Autodesk Inventor part; units mm, degrees
(part 4 of 4)
  line L290 (119.5666, 122.9451) -> (119.5666, 123.8935)
  line L291 (119.5666, 123.8935) -> (127.8065, 123.8935)
  line L292 (127.8065, 123.8935) -> (127.8065, 125.5163)
  line L293 (127.8065, 125.5163) -> (128.7402, 125.5163)
  line L294 (128.7402, 126.4722) -> (119.5962, 129.5548)
  line L295 (119.5962, 129.5548) -> (119.5962, 131.0516)
  line L296 (119.5962, 131.0516) -> (128.7402, 134.1342)
  line L297 (128.7402, 134.1342) -> (128.7402, 132.8523)
  line L298 (128.7402, 132.8523) -> (126.1837, 132.0224)
  line L299 (126.1837, 132.0224) -> (126.1837, 128.5322)
  line L300 (126.1837, 128.5322) -> (128.7402, 127.7023)
  line L301 (128.7402, 127.7023) -> (128.7402, 126.4722)
  line L302 (125.1463, 131.6889) -> (120.8411, 130.2736)
  line L303 (120.8411, 130.2736) -> (125.1463, 128.8657)
  line L304 (125.1463, 128.8657) -> (125.1463, 131.6889)
  spline S260 degree 2 poles (128.9032, 141.4776) (128.9032, 140.4846) (128.4883, 139.0916) (128.1919, 138.4765) knots 0 0 0 1 2 2 2
  line L305 (128.1919, 138.4765) -> (126.6654, 138.4765)
  line L306 (126.6654, 138.4765) -> (126.6654, 138.5654)
  spline S261 degree 2 poles (126.6654, 138.5654) (127.2286, 139.1657) (127.851, 140.6847) (127.851, 141.3887) knots 0 0 0 1 2 2 2
  spline S262 degree 2 poles (127.851, 141.3887) (127.851, 142.3964) (127.0137, 143.4264) (126.3245, 143.4264) knots 0 0 0 1 2 2 2
  spline S263 degree 2 poles (126.3245, 143.4264) (125.7762, 143.4264) (125.0945, 142.8855) (124.924, 142.3001) knots 0 0 0 1 2 2 2
  spline S264 degree 2 poles (124.924, 142.3001) (124.8055, 141.8777) (124.6425, 141.1738) (124.5091, 140.6477) knots 0 0 0 1 2 2 2
  spline S265 degree 2 poles (124.5091, 140.6477) (124.3831, 140.1734) (124.0052, 139.425) (123.7014, 139.136) knots 0 0 0 1 2 2 2
  spline S266 degree 2 poles (123.7014, 139.136) (123.3976, 138.8544) (122.5825, 138.5432) (122.0489, 138.5432) knots 0 0 0 1 2 2 2
  spline S267 degree 2 poles (122.0489, 138.5432) (120.9374, 138.5432) (119.4332, 140.2772) (119.4332, 141.6184) knots 0 0 0 1 2 2 2
  spline S268 degree 2 poles (119.4332, 141.6184) (119.4332, 142.389) (119.737, 143.7525) (120.026, 144.3379) knots 0 0 0 1 2 2 2
  line L307 (120.026, 144.3379) -> (121.4784, 144.3379)
  line L308 (121.4784, 144.3379) -> (121.4784, 144.2489)
  spline S269 degree 2 poles (121.4784, 144.2489) (121.0782, 143.8118) (120.4854, 142.4483) (120.4854, 141.6999) knots 0 0 0 1 2 2 2
  spline S270 degree 2 poles (120.4854, 141.6999) (120.4854, 140.8551) (121.2783, 139.8103) (121.923, 139.8103) knots 0 0 0 1 2 2 2
  spline S271 degree 2 poles (121.923, 139.8103) (122.5009, 139.8103) (123.1901, 140.4254) (123.3457, 141.0033) knots 0 0 0 1 2 2 2
  spline S272 degree 2 poles (123.3457, 141.0033) (123.4494, 141.3887) (123.7162, 142.5076) (123.8273, 142.8781) knots 0 0 0 1 2 2 2
  spline S273 degree 2 poles (123.8273, 142.8781) (124.1163, 143.8192) (125.2797, 144.6935) (126.1319, 144.6935) knots 0 0 0 1 2 2 2
  spline S274 degree 2 poles (126.1319, 144.6935) (126.6728, 144.6935) (127.7102, 144.2564) (128.0733, 143.8636) knots 0 0 0 1 2 2 2
  spline S275 degree 2 poles (128.0733, 143.8636) (128.4734, 143.4264) (128.9032, 142.3149) (128.9032, 141.4776) knots 0 0 0 1 2 2 2
  line L309 (128.7402, 145.931) -> (119.5962, 145.931)
  line L310 (119.5962, 145.931) -> (119.5962, 151.6516)
  line L311 (119.5962, 151.6516) -> (120.6781, 151.6516)
  line L312 (120.6781, 151.6516) -> (120.6781, 147.1463)
  line L313 (120.6781, 147.1463) -> (123.1827, 147.1463)
  line L314 (123.1827, 147.1463) -> (123.1827, 151.3478)
  line L315 (123.1827, 151.3478) -> (124.2645, 151.3478)
  line L316 (124.2645, 151.3478) -> (124.2645, 147.1463)
  line L317 (124.2645, 147.1463) -> (127.6583, 147.1463)
  line L318 (127.6583, 147.1463) -> (127.6583, 151.6516)
  line L319 (127.6583, 151.6516) -> (128.7402, 151.6516)
  line L320 (128.7402, 151.6516) -> (128.7402, 145.931)
  spline S276 degree 2 poles (128.9032, 156.557) (128.9032, 155.6678) (128.303, 154.1636) (127.7028, 153.6152) knots 0 0 0 1 2 2 2
  spline S277 degree 2 poles (127.7028, 153.6152) (127.11, 153.0669) (125.3316, 152.4667) (124.1756, 152.4667) knots 0 0 0 1 2 2 2
  spline S278 degree 2 poles (124.1756, 152.4667) (123.0271, 152.4667) (121.3228, 153.0521) (120.6929, 153.6078) knots 0 0 0 1 2 2 2
  spline S279 degree 2 poles (120.6929, 153.6078) (120.0779, 154.1562) (119.4332, 155.653) (119.4332, 156.5793) knots 0 0 0 1 2 2 2
  spline S280 degree 2 poles (119.4332, 156.5793) (119.4332, 157.0387) (119.5666, 157.8464) (119.6703, 158.1872) knots 0 0 0 1 2 2 2
  spline S281 degree 2 poles (119.6703, 158.1872) (119.7666, 158.4836) (120.0408, 159.0987) (120.2038, 159.4025) knots 0 0 0 1 2 2 2
  line L321 (120.2038, 159.4025) -> (121.671, 159.4025)
  line L322 (121.671, 159.4025) -> (121.671, 159.3062)
  spline S282 degree 2 poles (121.671, 159.3062) (121.5228, 159.1431) (121.1079, 158.6393) (120.9078, 158.2762) knots 0 0 0 1 2 2 2
  spline S283 degree 2 poles (120.9078, 158.2762) (120.7151, 157.9279) (120.4706, 157.1054) (120.4706, 156.5719) knots 0 0 0 1 2 2 2
  spline S284 degree 2 poles (120.4706, 156.5719) (120.4706, 155.9865) (120.9522, 154.9416) (121.4117, 154.5489) knots 0 0 0 1 2 2 2
  spline S285 degree 2 poles (121.4117, 154.5489) (121.8785, 154.1636) (123.2938, 153.7338) (124.1756, 153.7338) knots 0 0 0 1 2 2 2
  spline S286 degree 2 poles (124.1756, 153.7338) (125.1167, 153.7338) (126.4727, 154.1858) (126.9396, 154.5786) knots 0 0 0 1 2 2 2
  spline S287 degree 2 poles (126.9396, 154.5786) (127.3916, 154.9639) (127.851, 155.9939) (127.851, 156.5719) knots 0 0 0 1 2 2 2
  spline S288 degree 2 poles (127.851, 156.5719) (127.851, 157.098) (127.5917, 157.9946) (127.399, 158.3429) knots 0 0 0 1 2 2 2
  spline S289 degree 2 poles (127.399, 158.3429) (127.2063, 158.6763) (126.8062, 159.1728) (126.6654, 159.3136) knots 0 0 0 1 2 2 2
  line L323 (126.6654, 159.3136) -> (126.6654, 159.4025)
  line L324 (126.6654, 159.4025) -> (128.1178, 159.4025)
  spline S290 degree 2 poles (128.1178, 159.4025) (128.2586, 159.0987) (128.5179, 158.5652) (128.6365, 158.1872) knots 0 0 0 1 2 2 2
  spline S291 degree 2 poles (128.6365, 158.1872) (128.7699, 157.7871) (128.9032, 157.1054) (128.9032, 156.557) knots 0 0 0 1 2 2 2
  line L325 (128.7402, 162.6703) -> (120.6781, 162.6703)
  line L326 (120.6781, 162.6703) -> (120.6781, 159.6026)
  line L327 (120.6781, 159.6026) -> (119.5962, 159.6026)
  line L328 (119.5962, 159.6026) -> (119.5962, 166.9533)
  line L329 (119.5962, 166.9533) -> (120.6781, 166.9533)
  line L330 (120.6781, 166.9533) -> (120.6781, 163.8856)
  line L331 (120.6781, 163.8856) -> (128.7402, 163.8856)
  line L332 (128.7402, 163.8856) -> (128.7402, 162.6703)
  line L333 (128.7402, 171.0659) -> (128.7402, 167.5239)
  line L334 (128.7402, 167.5239) -> (127.8065, 167.5239)
  line L335 (127.8065, 167.5239) -> (127.8065, 168.6873)
  line L336 (127.8065, 168.6873) -> (120.5299, 168.6873)
  line L337 (120.5299, 168.6873) -> (120.5299, 167.5239)
  line L338 (120.5299, 167.5239) -> (119.5962, 167.5239)
  line L339 (119.5962, 167.5239) -> (119.5962, 171.0659)
  line L340 (119.5962, 171.0659) -> (120.5299, 171.0659)
  line L341 (120.5299, 171.0659) -> (120.5299, 169.9025)
  line L342 (120.5299, 169.9025) -> (127.8065, 169.9025)
  line L343 (127.8065, 169.9025) -> (127.8065, 171.0659)
  line L344 (127.8065, 171.0659) -> (128.7402, 171.0659)
  spline S292 degree 2 poles (120.641, 179.0391) (121.2487, 179.5578) (123.0271, 180.1358) (124.1682, 180.1358) knots 0 0 0 1 2 2 2
  spline S293 degree 2 poles (124.1682, 180.1358) (125.2797, 180.1358) (127.0804, 179.5726) (127.688, 179.0391) knots 0 0 0 1 2 2 2
  spline S294 degree 2 poles (127.688, 179.0391) (128.3252, 178.476) (128.9329, 176.9865) (128.9329, 176.0899) knots 0 0 0 1 2 2 2
  spline S295 degree 2 poles (128.9329, 176.0899) (128.9329, 175.1637) (128.303, 173.6817) (127.688, 173.1407) knots 0 0 0 1 2 2 2
  spline S296 degree 2 poles (127.688, 173.1407) (127.0804, 172.6146) (125.2945, 172.0514) (124.1682, 172.0514) knots 0 0 0 1 2 2 2
  spline S297 degree 2 poles (124.1682, 172.0514) (123.0197, 172.0514) (121.2709, 172.622) (120.641, 173.1481) knots 0 0 0 1 2 2 2
  spline S298 degree 2 poles (120.641, 173.1481) (120.0334, 173.6817) (119.4035, 175.1711) (119.4035, 176.0899) knots 0 0 0 1 2 2 2
  spline S299 degree 2 poles (119.4035, 176.0899) (119.4035, 177.0236) (120.0556, 178.5204) (120.641, 179.0391) knots 0 0 0 1 2 2 2
  spline S300 degree 2 poles (124.1682, 178.8687) (123.2642, 178.8687) (121.8637, 178.476) (121.4043, 178.1203) knots 0 0 0 1 2 2 2
  spline S301 degree 2 poles (121.4043, 178.1203) (120.93, 177.7572) (120.4558, 176.7346) (120.4558, 176.0973) knots 0 0 0 1 2 2 2
  spline S302 degree 2 poles (120.4558, 176.0973) (120.4558, 175.4378) (120.9152, 174.4449) (121.4043, 174.067) knots 0 0 0 1 2 2 2
  spline S303 degree 2 poles (121.4043, 174.067) (121.8711, 173.7039) (123.279, 173.3186) (124.1682, 173.3186) knots 0 0 0 1 2 2 2
  spline S304 degree 2 poles (124.1682, 173.3186) (125.9689, 173.3186) (127.8806, 174.8302) (127.8806, 176.0973) knots 0 0 0 1 2 2 2
  spline S305 degree 2 poles (127.8806, 176.0973) (127.8806, 177.3645) (125.9689, 178.8687) (124.1682, 178.8687) knots 0 0 0 1 2 2 2
  line L345 (128.7402, 188.0127) -> (128.7402, 186.6492)
  line L346 (128.7402, 186.6492) -> (120.8559, 182.6034)
  line L347 (120.8559, 182.6034) -> (128.7402, 182.6034)
  line L348 (128.7402, 182.6034) -> (128.7402, 181.4696)
  line L349 (128.7402, 181.4696) -> (119.5962, 181.4696)
  line L350 (119.5962, 181.4696) -> (119.5962, 183.1962)
  line L351 (119.5962, 183.1962) -> (126.8358, 186.879)
  line L352 (126.8358, 186.879) -> (119.5962, 186.879)
  line L353 (119.5962, 186.879) -> (119.5962, 188.0127)
  line L354 (119.5962, 188.0127) -> (128.7402, 188.0127)
  spline S306 degree 2 poles (125.9318, 199.9947) (126.6135, 199.9947) (127.6583, 199.476) (127.9992, 199.0463) knots 0 0 0 1 2 2 2
  spline S307 degree 2 poles (127.9992, 199.0463) (128.3993, 198.5276) (128.7402, 197.3494) (128.7402, 196.4157) knots 0 0 0 1 2 2 2
  line L355 (128.7402, 196.4157) -> (128.7402, 193.7925)
  line L356 (128.7402, 193.7925) -> (119.5962, 193.7925)
  line L357 (119.5962, 193.7925) -> (119.5962, 196.2156)
  spline S308 degree 2 poles (119.5962, 196.2156) (119.5962, 197.1937) (119.7222, 198.1719) (119.9667, 198.6165) knots 0 0 0 1 2 2 2
  spline S309 degree 2 poles (119.9667, 198.6165) (120.2261, 199.1129) (121.0782, 199.565) (121.6562, 199.565) knots 0 0 0 1 2 2 2
  spline S310 degree 2 poles (121.6562, 199.565) (122.3009, 199.565) (123.3235, 198.8832) (123.6125, 198.283) knots 0 0 0 1 2 2 2
  line L358 (123.6125, 198.283) -> (123.6569, 198.283)
  spline S311 degree 2 poles (123.6569, 198.283) (123.8792, 199.0981) (125.0574, 199.9947) (125.9318, 199.9947) knots 0 0 0 1 2 2 2
  spline S312 degree 2 poles (125.9837, 198.7276) (125.465, 198.7276) (124.7981, 198.4312) (124.5609, 197.9866) knots 0 0 0 1 2 2 2
  spline S313 degree 2 poles (124.5609, 197.9866) (124.4127, 197.6976) (124.3238, 197.0159) (124.3238, 196.386) knots 0 0 0 1 2 2 2
  line L359 (124.3238, 196.386) -> (124.3238, 195.0078)
  line L360 (124.3238, 195.0078) -> (127.7028, 195.0078)
  line L361 (127.7028, 195.0078) -> (127.7028, 195.9933)
  spline S314 degree 2 poles (127.7028, 195.9933) (127.7028, 196.7936) (127.5546, 197.7124) (127.3175, 198.0681) knots 0 0 0 1 2 2 2
  spline S315 degree 2 poles (127.3175, 198.0681) (127.0729, 198.409) (126.4653, 198.7276) (125.9837, 198.7276) knots 0 0 0 1 2 2 2
  spline S316 degree 2 poles (121.8266, 198.2978) (121.5006, 198.2978) (121.0115, 198.0755) (120.8707, 197.831) knots 0 0 0 1 2 2 2
  spline S317 degree 2 poles (120.8707, 197.831) (120.7077, 197.5346) (120.6336, 196.8158) (120.6336, 196.1712) knots 0 0 0 1 2 2 2
  line L362 (120.6336, 196.1712) -> (120.6336, 195.0078)
  line L363 (120.6336, 195.0078) -> (123.3086, 195.0078)
  line L364 (123.3086, 195.0078) -> (123.3086, 196.386)
  spline S318 degree 2 poles (123.3086, 196.386) (123.3086, 196.9566) (123.1901, 197.4976) (123.0048, 197.7865) knots 0 0 0 1 2 2 2
  spline S319 degree 2 poles (123.0048, 197.7865) (122.827, 198.0681) (122.2564, 198.2978) (121.8266, 198.2978) knots 0 0 0 1 2 2 2
  spline S320 degree 2 poles (124.1682, 206.6341) (126.6283, 206.6341) (128.9329, 205.204) (128.9329, 203.7146) knots 0 0 0 1 2 2 2
  spline S321 degree 2 poles (128.9329, 203.7146) (128.9329, 202.2029) (126.5839, 200.7876) (124.1756, 200.7876) knots 0 0 0 1 2 2 2
  spline S322 degree 2 poles (124.1756, 200.7876) (121.7007, 200.7876) (119.411, 202.2178) (119.411, 203.7146) knots 0 0 0 1 2 2 2
  spline S323 degree 2 poles (119.411, 203.7146) (119.411, 205.2188) (121.7822, 206.6341) (124.1682, 206.6341) knots 0 0 0 1 2 2 2
  spline S324 degree 2 poles (126.9544, 205.0632) (126.5024, 205.2411) (125.1093, 205.3893) (124.1682, 205.3893) knots 0 0 0 1 2 2 2
  spline S325 degree 2 poles (124.1682, 205.3893) (123.2271, 205.3893) (121.8415, 205.2411) (121.3746, 205.0558) knots 0 0 0 1 2 2 2
  spline S326 degree 2 poles (121.3746, 205.0558) (120.9078, 204.8706) (120.4261, 204.2259) (120.4261, 203.7146) knots 0 0 0 1 2 2 2
  spline S327 degree 2 poles (120.4261, 203.7146) (120.4261, 203.2033) (120.9078, 202.5438) (121.3894, 202.3511) knots 0 0 0 1 2 2 2
  spline S328 degree 2 poles (121.3894, 202.3511) (121.8563, 202.1659) (123.279, 202.0325) (124.1756, 202.0325) knots 0 0 0 1 2 2 2
  spline S329 degree 2 poles (124.1756, 202.0325) (125.1389, 202.0325) (126.4283, 202.1511) (126.9322, 202.3437) knots 0 0 0 1 2 2 2
  spline S330 degree 2 poles (126.9322, 202.3437) (127.4064, 202.5216) (127.9177, 203.1811) (127.9177, 203.7146) knots 0 0 0 1 2 2 2
  spline S331 degree 2 poles (127.9177, 203.7146) (127.9177, 204.2185) (127.436, 204.878) (126.9544, 205.0632) knots 0 0 0 1 2 2 2
  spline S332 degree 2 poles (120.4632, 210.2725) (120.4632, 209.939) (120.6262, 209.2795) (120.7522, 208.9609) knots 0 0 0 1 2 2 2
  spline S333 degree 2 poles (120.7522, 208.9609) (120.8781, 208.6645) (121.1449, 208.2273) (121.2635, 208.0569) knots 0 0 0 1 2 2 2
  line L365 (121.2635, 208.0569) -> (121.2635, 207.9828)
  line L366 (121.2635, 207.9828) -> (119.9667, 207.9828)
  spline S334 degree 2 poles (119.9667, 207.9828) (119.7518, 208.3829) (119.4035, 209.7538) (119.4035, 210.3688) knots 0 0 0 1 2 2 2
  spline S335 degree 2 poles (119.4035, 210.3688) (119.4035, 210.9913) (119.6555, 211.9175) (119.9223, 212.2954) knots 0 0 0 1 2 2 2
  spline S336 degree 2 poles (119.9223, 212.2954) (120.2112, 212.6956) (121.0486, 213.1105) (121.6117, 213.1105) knots 0 0 0 1 2 2 2
  spline S337 degree 2 poles (121.6117, 213.1105) (122.3676, 213.1105) (123.5087, 212.1176) (123.6569, 211.421) knots 0 0 0 1 2 2 2
  line L367 (123.6569, 211.421) -> (123.7458, 211.421)
  spline S338 degree 2 poles (123.7458, 211.421) (123.8051, 211.71) (124.0719, 212.3695) (124.3386, 212.6511) knots 0 0 0 1 2 2 2
  spline S339 degree 2 poles (124.3386, 212.6511) (124.598, 212.9327) (125.4279, 213.2884) (126.0281, 213.2884) knots 0 0 0 1 2 2 2
  spline S340 degree 2 poles (126.0281, 213.2884) (126.6432, 213.2884) (127.688, 212.866) (128.0881, 212.4807) knots 0 0 0 1 2 2 2
  spline S341 degree 2 poles (128.0881, 212.4807) (128.5031, 212.0805) (128.9329, 210.9468) (128.9329, 210.228) knots 0 0 0 1 2 2 2
  spline S342 degree 2 poles (128.9329, 210.228) (128.9329, 209.5389) (128.5994, 208.1903) (128.3697, 207.7308) knots 0 0 0 1 2 2 2
  line L368 (128.3697, 207.7308) -> (127.0729, 207.7308)
  line L369 (127.0729, 207.7308) -> (127.0729, 207.8198)
  spline S343 degree 2 poles (127.0729, 207.8198) (127.3545, 208.2051) (127.8732, 209.5092) (127.8732, 210.1539) knots 0 0 0 1 2 2 2
  spline S344 degree 2 poles (127.8732, 210.1539) (127.8732, 210.5318) (127.6361, 211.2877) (127.3619, 211.5396) knots 0 0 0 1 2 2 2
  spline S345 degree 2 poles (127.3619, 211.5396) (127.0878, 211.7841) (126.4357, 212.0435) (125.9392, 212.0435) knots 0 0 0 1 2 2 2
  spline S346 degree 2 poles (125.9392, 212.0435) (125.4427, 212.0435) (124.7981, 211.7545) (124.6128, 211.4951) knots 0 0 0 1 2 2 2
  spline S347 degree 2 poles (124.6128, 211.4951) (124.4276, 211.2358) (124.2868, 210.5318) (124.2868, 210.1169) knots 0 0 0 1 2 2 2
  line L370 (124.2868, 210.1169) -> (124.2868, 209.5982)
  line L371 (124.2868, 209.5982) -> (123.2716, 209.5982)
  line L372 (123.2716, 209.5982) -> (123.2716, 210.0057)
  spline S348 degree 2 poles (123.2716, 210.0057) (123.2716, 210.8282) (122.4861, 211.8656) (121.7377, 211.8656) knots 0 0 0 1 2 2 2
  spline S349 degree 2 poles (121.7377, 211.8656) (121.3894, 211.8656) (120.893, 211.5989) (120.7448, 211.384) knots 0 0 0 1 2 2 2
  spline S350 degree 2 poles (120.7448, 211.384) (120.5892, 211.1543) (120.4632, 210.5911) (120.4632, 210.2725) knots 0 0 0 1 2 2 2
  dimension "d91" = 304.8
  dimension "d92" = 203.2
  dimension "d93" = 127
  dimension "d94" = 101.6
  dimension "d95" = 50.8
  dimension "d96" = 88.9
  constraints: 2 other
  measures "d91" distance of L1.end L2.end
  measures "d92" distance of L2.end L0.start
  measures "d93" distance of L4.start L4.end
  measures "d94" distance of L6.end L4.start
  measures "d95" distance between parallel lines of L0 L6
  measures "d96" distance between parallel lines of L3 L7
extrude "Extrusion6" cut sketch "Sketch6" against normal blind 5.08 contours S0 S1 L8 L9 S2 S3 S4 L10 L11 L12 L13 L14 | S5 S6 L15 L16 L17 S7 S8 S9 S10 L18 L19 L20 S11 S12 | S13 L21 L22 S14 S15 S16 S17 S18 S19 S20 S21 L23 L24 S22 S23 S24 S25 S26 S27 S28 | L25 L26 L27 L28 L29 L30 L31 L32 | L33 L34 L35 L36 L37 L38 L39 L40 L41 L42 L43 L44 | L45 L46 L47 L48 L49 L50 L51 L52 L53 L54 | L55 L56 L57 L58 L59 L60 L61 L62 | L66 L67 L68 L69 L70 L71 | L72 L73 L74 L75 L76 L77 | L78 L79 L80 L81 L82 L83 L84 L85 L86 L87 L88 L89 | L90 L91 L92 L93 L94 L95 L96 L97 L98 L99 | L100 L101 L102 L103 L104 L105 L106 L107 | L111 L112 L113 L114 L115 L116 S29 L117 L118 L119 L120 | L121 L122 L123 L124 L125 L126 L127 L128 L129 L130 L131 | S30 S31 S32 L135 L136 S33 S34 S35 S36 S37 S38 S39 L137 L138 L139 L140 L141 S40 S41 S42 | S43 S44 S45 S46 S47 S48 S49 L142 L143 S50 S51 S52 S53 S54 | S62 S63 S64 S65 S66 S67 S68 L144 L145 S69 S70 S71 S72 S73 | S81 S82 S83 S84 | L146 L147 L148 L149 L150 L151 L152 | L153 L154 L155 L156 L157 L158 S93 L159 L160 L161 L162 | S94 S95 L163 L164 S96 S97 S98 L165 L166 L167 L168 L169 | L170 L171 L172 L173 | S99 S100 L174 L175 L176 L177 L178 S101 S102 | S107 S108 S109 S110 S111 S112 L180 S113 S114 S115 L181 L182 S116 S117 S118 L183 L184 L185 | L187 L188 L189 L190 | L191 L192 L193 L194 | S123 S124 S125 S126 L195 L196 S127 S128 S129 L197 L198 S130 S131 | L200 L201 S136 S137 S138 L202 L203 L204 L205 L206 S139 S140 L207 | S141 L208 L209 S142 S143 S144 S145 L210 L211 L212 L213 S146 S147 S148 S149 S150 L214 S151 S152 S153 S154 | L216 L217 S159 S160 S161 L218 L219 L220 S162 S163 S164 L221 L222 L223 | S165 S166 S167 S168 S169 L224 L225 S170 S171 S172 S173 S174 L226 L227 S175 S176 | S177 L228 L229 S178 S179 S180 S181 S182 S183 S184 S185 S186 L230 L231 S187 S188 S189 S190 S191 S192 S193 | L232 L233 S194 S195 S196 S197 S198 S199 S200 L234 L235 L236 | L238 L239 L240 L241 | S205 S206 S207 S208 L242 L243 S209 S210 S211 L244 L245 S212 S213 | L247 L248 S218 S219 S220 S221 S222 S223 S224 L249 L250 L251 | L253 L254 S229 S230 S231 L255 L256 L257 S232 S233 S234 L258 L259 L260 | L261 L262 L263 L264 L265 L266 L267 L268 L269 L270 L271 L272 L273 | S235 S236 L274 L275 L276 S237 S238 S239 S240 L277 L278 L279 S241 S242 | S243 L280 L281 S244 S245 S246 S247 S248 S249 S250 S251 L282 L283 S252 S253 S254 S255 S256 S257 S258 | L284 L285 L286 L287 L288 L289 S259 L290 L291 L292 L293 | L294 L295 L296 L297 L298 L299 L300 L301 | S260 L305 L306 S261 S262 S263 S264 S265 S266 S267 S268 L307 L308 S269 S270 S271 S272 S273 S274 S275 | L309 L310 L311 L312 L313 L314 L315 L316 L317 L318 L319 L320 | S276 S277 S278 S279 S280 S281 L321 L322 S282 S283 S284 S285 S286 S287 S288 S289 L323 L324 S290 S291 | L325 L326 L327 L328 L329 L330 L331 L332 | L333 L334 L335 L336 L337 L338 L339 L340 L341 L342 L343 L344 | S292 S293 S294 S295 S296 S297 S298 S299 | L345 L346 L347 L348 L349 L350 L351 L352 L353 L354 | S306 S307 L355 L356 L357 S308 S309 S310 L358 S311 | S320 S321 S322 S323 | S332 S333 L365 L366 S334 S335 S336 S337 L367 S338 S339 S340 S341 S342 L368 L369 S343 S344 S345 S346 S347 L370 L371 L372 S348 S349 S350
equation "\"d6\" = 0.5 * d2 - 0.5 * d4"
equation "\"d7\" = 0.5 * d3 - 0.5 * d5"
equation "\"d14\" = 0.5 * d10 - 0.5 * d12"
equation "\"d15\" = 0.5 * d11 - 0.5 * d13"
equation "\"d22\" = 0.5 * d19 - 0.5 * d18"
equation "\"d23\" = 0.5 * d20 - 0.5 * d21"
equation "\"d28\" = 0.75 * d27"
equation "\"d29\" = 0.5 * d27 - 0.5 * d28"
equation "\"d31\" = 0.0833333 * d26 - 0.5 * d30"
equation "\"d35\" = 0.5 * d27 - 0.5 * d33"
equation "\"d36\" = 0.5 * d32 - 0.5 * d34"
equation "\"d39\" = 0.0833333 * d26"
equation "\"d44\" = d33"
equation "\"d45\" = d34"
equation "\"d47\" = 0.0833333 * d26"
equation "\"d48\" = d35"
equation "\"d49\" = d45"
equation "\"d50\" = d45"
equation "\"d51\" = d35"
equation "\"d52\" = d47"
equation "\"d53\" = d49"
equation "\"d54\" = d50"
equation "\"d55\" = d35"
equation "\"d56\" = d47"
equation "\"d57\" = d49"
equation "\"d58\" = d50"
equation "\"d59\" = d35"
equation "\"d60\" = d47"
body "Solid1"
